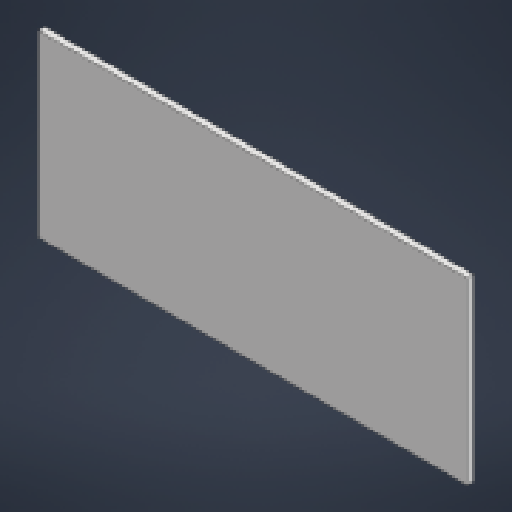
# Autodesk Inventor part: 挡板
Saved by Autodesk Inventor 2025 (Build 290162000, 162)
## iProperties
Created: 2024-12-26
Part Number: 挡板
Material: 常规
Document SubType Name: Modeling
Designer: HZD
Density: 1 g/cm^3
Appearance: 默认
Author: HZD
Autodesk Inventor part; units mm, degrees
ref_plane "YZ Plane" through (0, 0, 0) normal (1, 0, 0) x (0, 1, 0)
ref_plane "XZ Plane" through (0, 0, 0) normal (0, 1, 0) x (-1, 0, 0)
ref_plane "XY Plane" through (0, 0, 0) normal (0, 0, 1) x (1, 0, 0)
sketch "草图1" plane through (0, 0, 0) normal (0, 0, 1) x (1, 0, 0)
  line L0 (100, -41.8681) -> (-100, -41.8681)
  line L1 (-100, -41.8681) -> (-100, 41.8681)
  line L2 (-100, 41.8681) -> (100, 41.8681)
  line L3 (100, 41.8681) -> (100, -41.8681)
  line L4 (100, -41.8681) -> (-100, 41.8681) construction
  line L5 (-100, -41.8681) -> (100, 41.8681) construction
  point P0 (0, 0)
  dimension "d4" = 200
  constraints: 12 end point, 2 midpoint, 2 parallel, 1 horizontal, 1 perpendicular
  measures "d4" distance between parallel lines of L1 L3
extrude "拉伸1" add sketch "草图1" along normal blind 3
